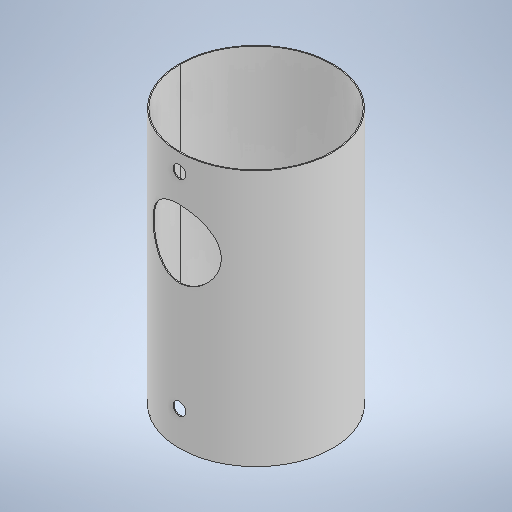
# Autodesk Inventor part: Стенка фильтра D1000
Saved by Autodesk Inventor 2025 (Build 290162010, 162A)
## iProperties
Created: 2025-02-11
Part Number: Стенка фильтра D1000
Material: Generic
Document SubType Name: Sheet Metal
Designer: pokla
Density: 1 g/cm^3
Appearance: Default
Flat Pattern Width: 160.4 cm
Flat Pattern Length: 299.713 cm
Flat Pattern Area: 48073.9 cm^2
Sheet Metal Rule: Default_mm
Sheet Metal Width: 1604,000 mm
Sheet Metal Length: 2997,126 mm
Sheet Metal Area: 4807390,539 mm^2
Author: pokla
Autodesk Inventor part; units mm, degrees
ref_plane "YZ Plane" through (0, 0, 0) normal (1, 0, 0) x (0, 1, 0)
ref_plane "XZ Plane" through (0, 0, 0) normal (0, 1, 0) x (-1, 0, 0)
ref_plane "XY Plane" through (0, 0, 0) normal (0, 0, 1) x (1, 0, 0)
sketch "Sketch1" plane through (0, 0, 0) normal (0, 1, 0) x (-1, 0, 0)
  line L0 (480.5, 1604) -> (474.5, 1604)
  line L1 (474.5, 1604) -> (474.5, 0)
  line L2 (474.5, 0) -> (480.5, 0)
  line L3 (480.5, 0) -> (480.5, 1604)
  line L4 (0, 0) -> (0, 1673.0415)
  point P0 (477.5, 0)
  dimension "d0" = 6
  dimension "d1" = 1604
  dimension "d2" = 949
  constraints: 10 end point, 2 parallel, 1 coincident, 1 horizontal, 1 horizontal alignment, 1 midpoint, 1 perpendicular, 1 vertical
  measures "d0" distance between parallel lines of L1 L3
  measures "d1" distance of L2.end L0.start
  measures "d2" diameter of L1 L4
revolve "Revolution1" add sketch "Sketch1" angle 359.9 about axis through (0, 0, 0) along (0, 0, 1)
sketch "Sketch2" plane through (0, 0, 0) normal (0, 1, 0) x (-1, 0, 0)
  circle A0 centre (0, 1109) radius 213
  circle A1 centre (0, 215) radius 40
  circle A2 centre (0, 1499) radius 40
  line L0 (474.5, 1604) -> (-474.5, 1604) projected
  point P0 (0, 0)
  point P1 (474.4993, 1604)
  dimension "d4" = 426
  dimension "d5" = 80
  dimension "d6" = 80
  dimension "d7" = 215
  dimension "d8" = 105
  dimension "d9" = 495
  constraints: 3 centre point, 3 vertical alignment
  measures "d4" diameter of A0
  measures "d5" diameter of A2
  measures "d6" diameter of A1
  measures "d7" distance of point (0, 0) A1.centre
  measures "d8" distance from line of L0 A2.centre
  measures "d9" distance from line of L0 A0.centre
extrude "Extrusion1" cut sketch "Sketch2" against normal through all
equation "\"d1\" = Высота_сред_части"
equation "\"d2\" = Внутр_Диам"
equation "\"d5\" = Внешний_диам_трубы_подкл"
equation "\"d6\" = Внешний_диам_трубы_подкл"
equation "\"BendRadius\" = Thickness"
equation "\"BendReliefWidth\" = Thickness"
equation "\"BendReliefDepth\" = 0.5 * Thickness"
equation "\"CornerReliefSize\" = 4 * Thickness"
equation "\"MinimumRemnant\" = 2 * Thickness"
equation "\"TransitionRadius\" = BendRadius"
equation "\"JacobiRadiusSize\" = BendRadius"
equation "\"GapSize\" = Thickness"
equation "\"Высота_сред_части\" = 1604"
equation "\"Внутр_Диам\" = 949"
equation "\"Внешний_диам_трубы_подкл\" = 80"
equation "\"Thickness\" = 6"
body "Solid1"
